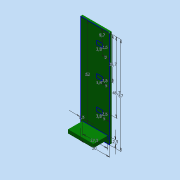
# Autodesk Inventor part: Sensor_Board_dummy
Saved by Autodesk Inventor 2015 (Build 190159000, 159)
## iProperties
Created: 2014-12-25
Part Number: Sensor_Board_dummy
Material: Generic
Document SubType Name: Modeling
Designer: Openlab
Density: 1 g/cm^3
Appearance: Dark Green
Author: Openlab
Autodesk Inventor part; units mm, degrees
ref_plane "YZ Plane" through (0, 0, 0) normal (1, 0, 0) x (0, 1, 0)
ref_plane "XZ Plane" through (0, 0, 0) normal (0, 1, 0) x (-1, 0, 0)
ref_plane "XY Plane" through (0, 0, 0) normal (0, 0, 1) x (1, 0, 0)
sketch "Sketch2" plane through (0, 0, 0) normal (0, 1, 0) x (-1, 0, 0)
  line L0 (20, 0) -> (0, 0)
  line L1 (0, 0) -> (0, -67)
  line L2 (0, -67) -> (20, -67)
  line L3 (20, -67) -> (20, 0)
  line L4 (18.5, -62) -> (1, -62)
  line L5 (1, -62) -> (1, -64.5)
  line L6 (1, -64.5) -> (18.5, -64.5)
  line L7 (18.5, -64.5) -> (18.5, -62)
  line L8 (8.8, -8.7) -> (5, -8.7)
  line L9 (5, -8.7) -> (5, -11.3)
  line L10 (5, -11.3) -> (8.8, -11.3)
  line L11 (8.8, -11.3) -> (8.8, -8.7)
  line L12 (8.8, -28.7) -> (5, -28.7)
  line L13 (5, -28.7) -> (5, -31.3)
  line L14 (5, -31.3) -> (8.8, -31.3)
  line L15 (8.8, -31.3) -> (8.8, -28.7)
  line L16 (8.8, -48.7) -> (5, -48.7)
  line L17 (5, -48.7) -> (5, -51.3)
  line L18 (5, -51.3) -> (8.8, -51.3)
  line L19 (8.8, -51.3) -> (8.8, -48.7)
  dimension "d0" = 20
  dimension "d1" = 67
  dimension "d2" = 17.5
  dimension "d3" = 2.5
  dimension "d4" = 1.5
  dimension "d6" = 8.7
  dimension "d9" = 3.8
  dimension "d10" = 2.6
  dimension "d11" = 3.8
  dimension "d12" = 2.6
  dimension "d13" = 3.8
  dimension "d14" = 2.6
  dimension "d16" = 28.7
  dimension "d17" = 48.7
  dimension "d18" = 62
  dimension "d27" = 5
  dimension "d28" = 5
  dimension "d29" = 5
  constraints: 40 end point, 10 parallel, 5 horizontal, 5 perpendicular, 1 coincident
  measures "d0" distance of L2.end L1.end
  measures "d1" distance of L1.end L0.end
  measures "d2" distance of L6.end L5.end
  measures "d3" distance of L5.end L4.end
  measures "d4" distance between parallel lines of L3 L7
  measures "d6" distance between parallel lines of L0 L8
  measures "d9" distance of L9.end L10.end
  measures "d10" distance of L8.end L9.end
  measures "d11" distance of L14.start L14.end
  measures "d12" distance of L13.start L14.start
  measures "d13" distance of L18.start L18.end
  measures "d14" distance of L17.start L18.start
  measures "d16" distance between parallel lines of L12 L0
  measures "d17" distance between parallel lines of L16 L0
  measures "d18" distance between parallel lines of L4 L0
  measures "d27" distance between parallel lines of L1 L9
  measures "d28" distance between parallel lines of L1 L13
  measures "d29" distance between parallel lines of L1 L17
extrude "Extrusion1" add sketch "Sketch2" along normal blind 1.5 contours L3 L2 L1 L0 | L7 L6 L5 L4 | L11 L10 L9 L8 | L15 L14 L13 L12 | L19 L18 L17 L16
extrude "Extrusion2" add sketch "Sketch2" along normal blind 2.85 contours L11 L10 L9 L8 | L15 L14 L13 L12 | L19 L18 L17 L16
extrude "Extrusion3" add sketch "Sketch2" against normal blind 10 contours L7 L6 L5 L4
body "Solid1"
